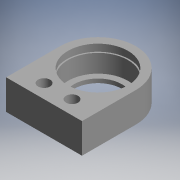
# Autodesk Inventor part: SBGSMA6200ZZ-20_h
Saved by Autodesk Inventor 2017.3 (Build 213256000, 256)
## iProperties
Part Number: SBGSMA6200ZZ-20_h
Material: Generic
Catalog Web Link: www.cadenas.de
Description: BGSMA, BGSMAB, SBGSMA_housing-Bearing with Housings - Front Installation Type
Vendor: MISUMI
Document SubType Name: Modeling
Designer: partserver
Manufacturer: MISUMI
Mass: 12.8727 g
Surface Area: 65.254 cm^2
Volume: 12.8727 cm^3
Density: 1 g/cm^3
Appearance: PSOLRGB-192-192-192
Category: PARTsolutions
Company: MISUMI
Title: SBGSMA6200ZZ-20
Author: Cadenas PARTsolutions
Comments: Bearing with Housings - Front Installation Type
PSOL_IDENT_0: {$CADENAS_DATA\23d-libs\misumi\metric\12_bearing_holders\bgsma\bgsma_housing.prj},218 {VTYP=3D},{NB=
PSOL_IDENT_1: SBGSMA6200ZZ-20_h},{LINA=SBGSMA6200ZZ-20},{NN=BGSMA, BGSMAB, SBGSMA_housing},{DATE=30.03.2018 01:48:
PSOL_IDENT_2: 31},{GEOMDATE=13.07.2015 10:26:00},{VERSION=},{LINEID=30},{WBVAR=MATB,STH,SEAL,HH,ALT1},{WBNUMERIC=H
PSOL_IDENT_3: H}  {NB=SBGSMA6200ZZ-20_h},{LINA=SBGSMA6200ZZ-20},{KT=DUMMY},{PN=SBGSMA6200ZZ-20},{TYPE=SBGSMA},{MAT
PSOL_IDENT_4: B=STS},{MATBALG= 'ST','Steel','STS','Stainless Steel' },{STH=},{STHALG= '','-' },{ARR=304 Stainless
PSOL_IDENT_5: Steel},{ARRALG=-S},{BN=6200},{SEAL=ZZ},{SEALALG= 'ZZ','ZZ(Double Shielded)','VV','VV(Non-contact Rub
PSOL_IDENT_6: ber Seal)','DD','DD(Contact Rubber Seal)' },{HH=20},{HHALG=20,25,30},{DD=10},{D=30},{DDHH=24},{B=9},
PSOL_IDENT_7: {H=46.0},{HH1=7},{L=38},{L1=14},{T=15},{DD1=6},{ALT1=},{ALT1ALG= '','Bearing and Retaining Ring Asse
PSOL_IDENT_8: mbled','NA','with NA (Bearing and Retaining Ring not Assembled)' },{ALT1PN=},{DD2=31.4},{TT=1.20}
NB: SBGSMA6200ZZ-20_h
NN: BGSMA, BGSMAB, SBGSMA_housing
NT: Bearing with Housings - Front Installation Type
NBSYN: $PN._h
LINA: SBGSMA6200ZZ-20
CATALOG: Misumi
PN: SBGSMA6200ZZ-20
MATB: Stainless Steel
STH: -
ARR: 304 Stainless Steel
BN: 6200
SEAL: ZZ(Double Shielded)
HH: 20
DD: 10
D: 30
DDHH: 24
B: 9
H: 46
HH1: 7
L: 38
L1: 14
T: 15
DD1: 6
ALT1: Bearing and Retaining Ring Assembled
SUPPLIER: MISUMI
ARTICLENO: SBGSMA6200ZZ-20_h
BOMINFO: SBGSMA6200ZZ-20
CREATOR: CADENAS GmbH
Autodesk Inventor part; units mm, degrees
sketch "Sketch_7" plane through (0, 0, 0) normal (0, 0, 1) x (1, 0, 0)
  line L0 (-19, 27) -> (-19, 0)
  line L1 (-19, 0) -> (19, 0)
  line L2 (19, 0) -> (19, 27)
  arc A0 (19, 27) -> (-19, 27) centre (0, 27) ccw
  constraints: 6 end point, 2 point on circle, 1 centre point
extrude "Extrusion1" add sketch "Sketch_7" against normal blind 15
sketch "Sketch_8" plane through (0, 0, 0) normal (1, 0, 0) x (0, 0, -1)
  line L0 (15, 27) -> (2, 27)
  line L1 (2, 27) -> (2, 42)
  line L2 (2, 42) -> (11, 42)
  line L3 (11, 42) -> (11, 42.7)
  line L4 (11, 42.7) -> (12.2, 42.7)
  line L5 (12.2, 42.7) -> (12.2, 42)
  line L6 (12.2, 42) -> (15, 42)
  line L7 (15, 42) -> (15, 27)
  line L8 (15, 27) -> (2, 27)
  constraints: 18 end point
revolve "Revolution1" cut sketch "Sketch_8" angle 360 about axis through (0, 27, -15) along (0, 0, -1)
sketch "Sketch_1" plane through (0, 0, 0) normal (1, 0, 0) x (0, 0, -1)
  line L0 (15, 27) -> (0, 27)
  line L1 (0, 27) -> (0, 39)
  line L2 (0, 39) -> (15, 39)
  line L3 (15, 39) -> (15, 27)
  line L4 (15, 27) -> (0, 27)
  constraints: 10 end point
revolve "Revolution2" cut sketch "Sketch_1" angle 360 about axis through (0, 27, -15) along (0, 0, -1)
sketch "Sketch4" plane through (0, 0, -15) normal (0, 0, -1) x (-1, 0, 0)
  point P0 (7, 7)
hole "Hole1" at (-7, 7, -15) direction (0, 0, 1) diameter 6 depth 15
pattern_linear "Rectangular Pattern1" count 2 spacing 14 along (1, 0, 0) of "Hole1"
ref_plane "to_bearing_XY" through (0, 27, -6.5) normal (0, 0, 1) x (1, 0, 0)
ref_plane "to_bearing_YZ" through (0, 27, -6.5) normal (1, 0, 0) x (0, 1, 0)
ref_plane "to_bearing_ZX" through (0, 27, -6.5) normal (0, 1, 0) x (0, 0, 1)
ref_plane "to_retaining_ring_XY" through (0, 27, -12.2) normal (0, 0, -1) x (1, 0, 0)
ref_plane "to_retaining_ring_YZ" through (0, 27, -12.2) normal (1, 0, 0) x (0, -1, 0)
ref_plane "to_retaining_ring_ZX" through (0, 27, -12.2) normal (0, -1, 0) x (0, 0, -1)
body "Solid1"
